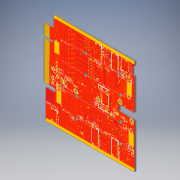
# Autodesk Inventor part: EPS_PCB
Saved by Autodesk Inventor 2018 (Build 220112000, 112)
## iProperties
Created: 2018-01-15
Part Number: EPS_PCB
Material: Epoxy Resin
Document SubType Name: Modeling
Designer: Bradley
Density: 1.14 g/cm^3
Appearance: Smooth - Medium Gray
Mass: 15.4834 g
Surface Area: 175.95 cm^2
Volume: 13.582 cm^3
Author: Bradley
Revision Number: 3.1
Autodesk Inventor part; units mm, degrees
ref_plane "YZ Plane" through (0, 0, 0) normal (1, 0, 0) x (0, 1, 0)
ref_plane "XZ Plane" through (0, 0, 0) normal (0, 1, 0) x (-1, 0, 0)
ref_plane "XY Plane" through (0, 0, 0) normal (0, 0, 1) x (1, 0, 0)
sketch "Sketch1" plane through (0, 0, 0) normal (0, 0, 1) x (1, 0, 0)
  line L0 (0, 36.15) -> (10, 36.15)
  line L1 (10, 36.15) -> (10, 47.9)
  line L2 (10, 47.9) -> (90.4, 47.9)
  line L3 (90.4, 47.9) -> (90.4, -47.9)
  line L4 (90.4, -47.9) -> (2, -47.9)
  line L5 (10, -15.15) -> (0, -15.15)
  line L6 (-5.5, 48) -> (90.5, 48) construction
  line L7 (90.5, 48) -> (90.5, -48) construction
  line L8 (90.5, -48) -> (-5.5, -48) construction
  line L9 (-5.5, -48) -> (-5.5, 48) construction
  line L10 (-5.4, 47.9) -> (-3.4, 47.9) construction
  line L11 (-3.4, 47.9) -> (-3.4, -47.9) construction
  line L12 (-3.4, -47.9) -> (-5.4, -47.9) construction
  line L13 (-5.4, -47.9) -> (-5.4, 47.9) construction
  line L14 (-3.4, 38.5) -> (7.85, 38.5) construction
  line L15 (7.85, 38.5) -> (7.85, -17.5) construction
  line L16 (7.85, -17.5) -> (-3.4, -17.5) construction
  line L17 (-3.4, -17.5) -> (-3.4, 38.5) construction
  line L18 (2, -47.9) -> (2, -18.65)
  line L19 (2, -18.65) -> (10, -18.65)
  arc A0 (10, -18.65) -> (10, -15.15) centre (10, -16.9) ccw
  line L20 (0, 24) -> (90.5, 24) construction
  circle A1 centre (-2.5, 47.1) radius 0.9 construction
  circle A2 centre (-0.7, 47.1) radius 0.9 construction
  circle A3 centre (1.1, 47.1) radius 0.9 construction
  circle A4 centre (2.9, 47.1) radius 0.9 construction
  circle A5 centre (4.7, 47.1) radius 0.9 construction
  circle A6 centre (6.5, 47.1) radius 0.9 construction
  circle A7 centre (8.3, 47.1) radius 0.9 construction
  circle A8 centre (-2.5, 45.3) radius 0.9 construction
  circle A9 centre (-0.7, 45.3) radius 0.9 construction
  circle A10 centre (1.1, 45.3) radius 0.9 construction
  circle A11 centre (2.9, 45.3) radius 0.9 construction
  circle A12 centre (4.7, 45.3) radius 0.9 construction
  circle A13 centre (6.5, 45.3) radius 0.9 construction
  circle A14 centre (8.3, 45.3) radius 0.9 construction
  circle A15 centre (-2.5, 43.5) radius 0.9 construction
  circle A16 centre (-0.7, 43.5) radius 0.9 construction
  circle A17 centre (1.1, 43.5) radius 0.9 construction
  circle A18 centre (2.9, 43.5) radius 0.9 construction
  circle A19 centre (4.7, 43.5) radius 0.9 construction
  circle A20 centre (6.5, 43.5) radius 0.9 construction
  circle A21 centre (8.3, 43.5) radius 0.9 construction
  circle A22 centre (-2.5, 41.7) radius 0.9 construction
  circle A23 centre (-0.7, 41.7) radius 0.9 construction
  circle A24 centre (1.1, 41.7) radius 0.9 construction
  circle A25 centre (2.9, 41.7) radius 0.9 construction
  circle A26 centre (4.7, 41.7) radius 0.9 construction
  circle A27 centre (6.5, 41.7) radius 0.9 construction
  circle A28 centre (8.3, 41.7) radius 0.9 construction
  circle A29 centre (-2.5, 39.9) radius 0.9 construction
  circle A30 centre (-0.7, 39.9) radius 0.9 construction
  circle A31 centre (1.1, 39.9) radius 0.9 construction
  circle A32 centre (2.9, 39.9) radius 0.9 construction
  circle A33 centre (4.7, 39.9) radius 0.9 construction
  circle A34 centre (6.5, 39.9) radius 0.9 construction
  circle A35 centre (8.3, 39.9) radius 0.9 construction
  line L21 (0, 36.15) -> (0, 24.95)
  line L22 (0, 24.95) -> (8.4, 24.95)
  arc A36 (8.4, 23.05) -> (8.4, 24.95) centre (8.4, 24) ccw
  line L23 (8.4, 23.05) -> (0, 23.05)
  line L24 (0, 23.05) -> (0, -15.15)
  point P0 (0, 0)
  point P1 (-5.5, 0)
  point P2 (90.4, 0)
  point P3 (90.5, 0)
  dimension "d0" = 51.3
  dimension "d1" = 95.8
  dimension "d3" = 10
  dimension "d20" = 96
  dimension "d21" = 96
  dimension "d22" = 0.1
  dimension "d23" = 0.1
  dimension "d24" = 2
  dimension "d25" = 0.1
  dimension "d28" = 11.25
  dimension "d29" = 56
  dimension "d31" = 9.5
  dimension "d32" = 30.5
  dimension "d34" = 3.5
  dimension "d35" = 12.15
  dimension "d36" = 39.15
  dimension "d37" = 14.5
  dimension "d38" = 1.15
  dimension "d39" = 1.8
  dimension "d42" = 1.8
  dimension "d45" = 1.8
  dimension "d48" = 2
  dimension "d49" = 3.4
  dimension "d50" = 1.9
  dimension "d51" = 8.4
  dimension "d52" = 24
  constraints: 50 end point, 37 centre point, 11 perpendicular, 7 parallel, 6 point on line, 6 tangent, 5 horizontal, 4 point on circle, 3 midpoint, 3 vertical, 2 collinear, 2 horizontal alignment, 68 other
  measures "d0" distance of L5.end L0.start
  measures "d1" distance of L2.end L3.end
  measures "d3" distance of L0.start L0.end
  measures "d20" distance of L6.start L6.end
  measures "d21" distance of L8.end L6.start
  measures "d22" distance between parallel lines of L2 L6
  measures "d23" distance between parallel lines of L7 L3
  measures "d24" distance between parallel lines of L13 L11
  measures "d25" distance between parallel lines of L13 L9
  measures "d28" distance of L15.end L16.end
  measures "d29" distance of L14.end L15.end
  measures "d31" distance between parallel lines of L14 L6
  measures "d32" distance between parallel lines of L8 L16
  measures "d34" distance between parallel lines of L5 L19
  measures "d35" distance between parallel lines of L20 L0
  measures "d36" distance between parallel lines of L5 L20
  measures "d37" distance between parallel lines of L20 L14
  measures "d38" distance between parallel lines of L19 L16
  measures "d39" diameter of A1
  measures "d42" distance of A1.centre A2.centre
  measures "d45" distance of A1.centre A8.centre
  measures "d48" distance between parallel lines of L18 L24
  measures "d49" distance between parallel lines of L24 L11
  measures "d50" distance between parallel lines of L23 L22
  measures "d51" distance of L21.end L22.end
  measures "d52" distance from line of point (0, 0) L20
extrude "Extrusion1" add sketch "Sketch1" along normal mid plane 1.6
chamfer "Chamfer1" distance 0.5 angle 45 4 edges at (0, 36.15, 0) (0, 24.95, 0) (0, 23.05, 0) (0, -15.15, 0)
fillet "Fillet1" radius 0.5 6 edges at (10, 36.15, 0) (10, 47.9, 0) (90.4, 47.9, 0) (90.4, -47.9, 0) (2, -47.9, 0) (2, -18.65, 0)
sketch "Sketch6" plane through (0, 0, 0.8) normal (0, 0, 1) x (1, 0, 0)
  arc A0 (2.5, -18.65) -> (2, -19.15) centre (2.5, -19.15) ccw projected
  line L0 (2, -19.15) -> (2, -47.4) projected
  arc A1 (2, -47.4) -> (2.5, -47.9) centre (2.5, -47.4) ccw projected
  line L1 (2.5, -47.9) -> (89.9, -47.9) projected
  arc A2 (89.9, -47.9) -> (90.4, -47.4) centre (89.9, -47.4) ccw projected
  line L2 (90.4, -47.4) -> (90.4, 47.4) projected
  arc A3 (90.4, 47.4) -> (89.9, 47.9) centre (89.9, 47.4) ccw projected
  line L3 (89.9, 47.9) -> (10.5, 47.9) projected
  arc A4 (10.5, 47.9) -> (10, 47.4) centre (10.5, 47.4) ccw projected
  line L4 (10, 47.4) -> (10, 36.65) projected
  arc A5 (9.5, 36.15) -> (10, 36.65) centre (9.5, 36.65) ccw projected
  line L5 (9.5, 36.15) -> (0.5, 36.15) projected
  line L6 (0, 35.65) -> (0.5, 36.15) projected
  line L7 (0, 35.65) -> (0, 25.45) projected
  line L8 (0.5, 24.95) -> (0, 25.45) projected
  line L9 (0.5, 24.95) -> (8.4, 24.95) projected
  arc A6 (8.4, 23.05) -> (8.4, 24.95) centre (8.4, 24) ccw projected
  line L10 (8.4, 23.05) -> (0.5, 23.05) projected
  line L11 (0, 22.55) -> (0.5, 23.05) projected
  line L12 (0, 22.55) -> (0, -14.65) projected
  line L13 (0.5, -15.15) -> (0, -14.65) projected
  line L14 (0.5, -15.15) -> (10, -15.15) projected
  arc A7 (10, -18.65) -> (10, -15.15) centre (10, -16.9) ccw projected
  line L15 (10, -18.65) -> (2.5, -18.65) projected
  line L16 (90.4, 47.4) -> (90.4, -47.4) projected
  arc A8 (89.4, 3) -> (90.4, 4) centre (89.4, 4) ccw
  line L17 (89.4, 3) -> (75.9, 3)
  arc A9 (75.9, 3) -> (74.9, 2) centre (75.9, 2) ccw
  line L18 (74.9, 2) -> (74.9, -2)
  arc A10 (74.9, -2) -> (75.9, -3) centre (75.9, -2) ccw
  line L19 (75.9, -3) -> (89.4, -3)
  arc A11 (90.4, -4) -> (89.4, -3) centre (89.4, -4) ccw
  arc A12 (90.4, 34) -> (89.4, 35) centre (89.4, 34) ccw
  arc A13 (88.4, 36) -> (89.4, 35) centre (89.4, 36) ccw
  line L20 (88.4, 36) -> (88.4, 42)
  arc A14 (89.4, 43) -> (88.4, 42) centre (89.4, 42) ccw
  arc A15 (89.4, 43) -> (90.4, 44) centre (89.4, 44) ccw
  point P0 (0, 0)
  point P1 (74.9, 0)
  dimension "d69" = 6
  dimension "d70" = 1
  dimension "d71" = 15.5
  dimension "d81" = 2
  dimension "d82" = 35
  dimension "d83" = 8
  constraints: 16 point on circle, 14 tangent, 8 centre point, 8 end point, 6 equal radius, 4 point on line, 2 perpendicular, 1 horizontal, 1 horizontal alignment, 1 midpoint, 1 vertical, 1 vertical alignment
  measures "d69" distance between parallel lines of L19 L17
  measures "d70" radius of A8
  measures "d71" distance between parallel lines of L2 L18
  measures "d81" distance between parallel lines of L16 L20
  measures "d82" vertical distance of point (0, 0) A12.end
  measures "d83" distance of A12.end A14.start
extrude "Extrusion5" cut sketch "Sketch6" against normal through all contours A11 L19 A10 L18 A9 L17 A8 L2 | A12 A13 L20 A14 A15 L2
sketch "Sketch14" plane through (0, 0, 0.8) normal (0, 0, 1) x (1, 0, 0)
  line L0 (0, 22.55) -> (0, -14.65) projected
  line L1 (90.4, 4) -> (90.4, 34) projected
  line L2 (0, 47.894) -> (90.4, 47.894) construction
  line L3 (90.4, 47.894) -> (90.4, -47.894) construction
  line L4 (90.4, -47.894) -> (0, -47.894) construction
  line L5 (0, -47.894) -> (0, 47.894) construction
  point P0 (0, 0)
  constraints: 1 collinear, 1 midpoint, 2 other
decal "Decal1"
sketch "Sketch15" plane through (0, 0, -0.8) normal (0, 0, -1) x (-1, 0, 0)
  line L0 (-90.4, 34) -> (-90.4, 4) projected
  line L1 (0, -14.65) -> (0, 22.55) projected
  line L2 (-90.4, 47.894) -> (0, 47.894) construction
  line L3 (0, 47.894) -> (0, -47.894) construction
  line L4 (0, -47.894) -> (-90.4, -47.894) construction
  line L5 (-90.4, -47.894) -> (-90.4, 47.894) construction
  point P0 (0, 0)
  constraints: 1 collinear, 1 midpoint, 2 other
decal "Decal2"
sketch "Sketch16" plane through (0, 0, 0.8) normal (0, 0, 1) x (1, 0, 0)
  point P0 (0, 0)
  point P1 (32.5, -11.5)
  point P2 (41.5, 30.5)
  point P3 (76, 30.5)
  point P4 (76, 11.5)
  point P5 (41.5, 11.5)
  point P6 (76, -11.5)
  point P7 (32.5, -30.5)
  point P8 (76, -30.5)
  constraints: 8 other
hole "Hole9" at (32.5, -11.5, 0.8) at (41.5, 30.5, 0.8) at (76, 30.5, 0.8) at (76, 11.5, 0.8) at (41.5, 11.5, 0.8) at (76, -11.5, 0.8) at (32.5, -30.5, 0.8) at (76, -30.5, 0.8) direction (0, 0, -1) diameter 3 end through all
sketch "Sketch17" plane through (0, 0, 0.8) normal (0, 0, 1) x (1, 0, 0)
  point P0 (0, 0)
  point P1 (75.9, 5.5)
  point P2 (54.3, -3.4)
  point P3 (87.4, -5.5)
  point P4 (31.9, -7.5)
  constraints: 4 other
hole "Hole10" at (75.9, 5.5, 0.8) at (54.3, -3.4, 0.8) at (87.4, -5.5, 0.8) at (31.9, -7.5, 0.8) direction (0, 0, -1) diameter 2.2 end through all
sketch "Sketch18" plane through (0, 0, 0.8) normal (0, 0, 1) x (1, 0, 0)
  point P0 (0, 0)
  point P1 (67.3, -9.5)
  point P2 (9.6, 0.7)
  point P3 (13.7, -4.1)
  point P4 (73.1, -5.9)
  constraints: 4 other
hole "Hole11" at (67.3, -9.5, 0.8) at (9.6, 0.7, 0.8) at (13.7, -4.1, 0.8) at (73.1, -5.9, 0.8) direction (0, 0, -1) diameter 1.5 end through all
sketch "Sketch19" plane through (0, 0, 0.8) normal (0, 0, 1) x (1, 0, 0)
  point P0 (0, 0)
  point P1 (57.46, 8)
  point P2 (62.54, 8)
  point P3 (62.54, -8)
  point P4 (57.46, -8)
  constraints: 4 other
hole "Hole12" at (57.46, 8, 0.8) at (62.54, 8, 0.8) at (62.54, -8, 0.8) at (57.46, -8, 0.8) direction (0, 0, -1) diameter 1.2 end through all
sketch "Sketch20" plane through (0, 0, 0.8) normal (0, 0, 1) x (1, 0, 0)
  point P0 (0, 0)
  point P1 (87.975, 4.15)
  point P2 (80.725, 4.15)
  point P3 (30.4, -3.2)
  constraints: 3 other
hole "Hole13" at (87.975, 4.15, 0.8) at (80.725, 4.15, 0.8) at (30.4, -3.2, 0.8) direction (0, 0, -1) diameter 0.7 end through all
sketch "Sketch21" plane through (0, 0, 0.8) normal (0, 0, 1) x (1, 0, 0)
  point P0 (0, 0)
  point P1 (74.769, 6.631)
  point P2 (74.3, 5.5)
  point P3 (74.769, 4.369)
  point P4 (75.9, 3.9)
  point P5 (77.031, 4.369)
  point P6 (89, -5.5)
  point P7 (88.531, -4.369)
  point P8 (86.269, -4.369)
  point P9 (30.769, -6.369)
  point P10 (30.3, -7.5)
  point P11 (30.769, -8.631)
  point P12 (31.9, -9.1)
  point P13 (33.031, -8.631)
  point P14 (88.531, -6.631)
  point P15 (55.9, -3.4)
  point P16 (55.431, -2.269)
  point P17 (54.3, -1.8)
  point P18 (53.169, -2.269)
  point P19 (52.7, -3.4)
  point P20 (87.4, -7.1)
  point P21 (54.3, -5)
  point P22 (55.431, -4.531)
  point P23 (33.5, -7.5)
  point P24 (33.031, -6.369)
  point P25 (31.9, -5.9)
  point P26 (87.4, -3.9)
  point P27 (77.5, 5.5)
  point P28 (77.031, 6.631)
  point P29 (75.9, 7.1)
  point P30 (86.269, -6.631)
  point P31 (85.8, -5.5)
  point P32 (53.169, -4.531)
  constraints: 32 other
hole "Hole14" at (74.769, 6.631, 0.8) at (74.3, 5.5, 0.8) at (74.769, 4.369, 0.8) at (75.9, 3.9, 0.8) at (77.031, 4.369, 0.8) at (89, -5.5, 0.8) at (88.531, -4.369, 0.8) at (86.269, -4.369, 0.8) at (30.769, -6.369, 0.8) at (30.3, -7.5, 0.8) at (30.769, -8.631, 0.8) at (31.9, -9.1, 0.8) at (33.031, -8.631, 0.8) at (88.531, -6.631, 0.8) at (55.9, -3.4, 0.8) at (55.431, -2.269, 0.8) at (54.3, -1.8, 0.8) at (53.169, -2.269, 0.8) at (52.7, -3.4, 0.8) at (87.4, -7.1, 0.8) at (54.3, -5, 0.8) at (55.431, -4.531, 0.8) at (33.5, -7.5, 0.8) at (33.031, -6.369, 0.8) at (31.9, -5.9, 0.8) at (87.4, -3.9, 0.8) at (77.5, 5.5, 0.8) at (77.031, 6.631, 0.8) at (75.9, 7.1, 0.8) at (86.269, -6.631, 0.8) at (85.8, -5.5, 0.8) at (53.169, -4.531, 0.8) direction (0, 0, -1) diameter 0.35 end through all
sketch "Sketch22" plane through (0, 0, 0.8) normal (0, 0, 1) x (1, 0, 0)
  point P0 (0, 0)
  point P1 (53.3, -21.6)
  point P2 (61.7, -27.3)
  point P3 (63.7, -24.1)
  point P4 (70.2, -35.2)
  point P5 (67.2, -35.2)
  point P6 (64.3, -35.2)
  point P7 (74.3, -34.5)
  point P8 (79.2, -31.9)
  point P9 (87.7, -11.7)
  point P10 (89.5, -7.5)
  point P11 (74.83, 21.6)
  point P12 (66.5, 32.5)
  point P13 (77, 26.5)
  point P14 (43.5, -36)
  point P15 (46.5, -36)
  point P16 (84, -31.5)
  point P17 (72.5, -26.5)
  point P18 (6, 13.5)
  point P19 (6, 12.5)
  point P20 (6, 11.5)
  point P21 (11.75, 44.15)
  point P22 (13.4, 40.05)
  point P23 (13.4, 35.95)
  point P24 (11.75, 31.7)
  point P25 (13.4, 11.35)
  point P26 (13.4, 7.25)
  point P27 (10.9, 2.25)
  point P28 (13.4, 15.35)
  point P29 (9.94, 19.885)
  point P30 (11.85, 26.56)
  point P31 (11.7, 29.55)
  point P32 (9.94, 21.51)
  point P33 (36.8, 43.65)
  point P34 (36.8, 6.85)
  point P35 (36.8, 15.25)
  point P36 (36.8, 19.15)
  point P37 (36.8, 23.25)
  point P38 (36.8, 27.35)
  point P39 (36.8, 31.45)
  point P40 (36.8, 35.55)
  point P41 (36.8, 39.65)
  point P42 (36.8, 10.95)
  point P43 (42.38, 43.68)
  point P44 (41.1, 38.3)
  point P45 (41.8, 35.5)
  point P46 (45.8, 43.7)
  point P47 (44.4, 41.1)
  point P48 (41.1, 41.1)
  point P49 (44.4, 38.3)
  point P50 (45.1, 35.5)
  point P51 (44.9, 26)
  point P52 (44.9, 23.2)
  point P53 (48.2, 26)
  point P54 (48.2, 23.2)
  point P55 (48.2, 20.4)
  point P56 (44.9, 20.4)
  point P57 (44.9, 17.6)
  point P58 (48.2, 17.6)
  point P59 (44.9, 14.8)
  point P60 (44.9, 12)
  point P61 (48.2, 12)
  point P62 (48.2, 14.8)
  point P63 (51.6, 42.7)
  point P64 (54.8, 22.2)
  point P65 (55.2, 25.6)
  point P66 (53.9, 30.9)
  point P67 (46.7, 35.5)
  point P68 (70, 43.8)
  point P69 (62.8, 43.8)
  point P70 (73.5, 33)
  point P71 (56.4, 43.8)
  point P72 (77.3, 43.8)
  point P73 (83.7, 43.8)
  point P74 (56.1, 33)
  point P75 (54.8, 15)
  point P76 (29.2, -11.9)
  point P77 (53, 0.9)
  point P78 (37.2, -16.9)
  point P79 (37.2, -17.6)
  point P80 (37.2, -18.3)
  point P81 (36.1, -9.8)
  point P82 (36.1, -10.6)
  point P83 (36.7, -4.5)
  point P84 (37.5, -4.5)
  point P85 (31.4, -2.5)
  point P86 (31.4, -3.9)
  point P87 (47.9, 1.5)
  point P88 (47.9, 2.2)
  point P89 (47.9, 0.8)
  point P90 (47.9, 0.1)
  point P91 (47.9, 2.9)
  point P92 (49.5, -7.2)
  point P93 (47.6, -9.1)
  point P94 (89.5, 7.1)
  point P95 (73.15, 1.2)
  point P96 (82.02, -6.1)
  point P97 (65.3, 9.1)
  point P98 (64.8, 13.6)
  point P99 (59.6, 12.4)
  point P100 (68.075, 9.1)
  point P101 (47.8, 7.6)
  point P102 (54.2, -42.5)
  point P103 (73.5, -40.5)
  point P104 (61.4, -42.7)
  point P105 (67.8, -42.7)
  point P106 (80.6, -42.6)
  point P107 (87.2, -42.3)
  point P108 (75.3, -38.1)
  point P109 (12.1, -41.3)
  point P110 (88.5, 9.7)
  point P111 (84.6, -3.9)
  point P112 (49.7, -18.8)
  point P113 (63.9, -16.1)
  point P114 (64.2, -18.8)
  point P115 (39, 6)
  point P116 (59.5, -8)
  point P117 (59, -3)
  point P118 (85, 39)
  point P119 (75.15, 23.135)
  point P120 (78.2, -34.2)
  point P121 (74.5, -33.75)
  point P122 (75.15, 22.375)
  point P123 (78.2, -35)
  point P124 (74.5, -35.25)
  point P125 (62.3, -1.2)
  point P126 (78.3, -20.9)
  point P127 (64.4, -11.5)
  point P128 (62.1, 42.2)
  point P129 (56.3, 40.5)
  point P130 (70.1, 42.2)
  point P131 (80.2, 39.6)
  point P132 (74.4, 42.5)
  point P133 (83, 39.6)
  point P134 (61.405, -44.41)
  point P135 (65.8, -35.2)
  point P136 (55, -44.1)
  point P137 (63, -35.2)
  point P138 (72.6, -43)
  point P139 (68.7, -35.2)
  point P140 (74.2, -43.1)
  point P141 (71.5, -35.2)
  point P142 (83.065, 30.67)
  point P143 (24.6, -40.3)
  point P144 (75.15, 23.895)
  point P145 (74.5, -32.2)
  point P146 (80.1, -33.1)
  point P147 (31.9, 20.8)
  point P148 (31.9, 24.9)
  point P149 (31.9, 29)
  point P150 (31.9, 33.1)
  point P151 (31.9, 37.2)
  point P152 (31.9, 41.3)
  point P153 (27.5, 43.095)
  point P154 (27.5, 39)
  point P155 (27.5, 34.9)
  point P156 (27.5, 30.8)
  point P157 (27.5, 26.7)
  point P158 (27.5, 22.6)
  point P159 (27.5, 18.5)
  point P160 (20.7, -14.4)
  point P161 (20.7, -11.3)
  point P162 (47.5, 37.6)
  point P163 (50.7, 17)
  point P164 (50.7, 9.8)
  point P165 (58.3, 33.7)
  point P166 (69.8, 38)
  point P167 (74.4, 25.6)
  point P168 (57.5, 26.7)
  point P169 (76.8, 34.7)
  point P170 (34.2, 2.5)
  point P171 (34.2, 1.9)
  point P172 (34.2, 1.2)
  point P173 (34.9, 1.2)
  point P174 (35.6, 1.2)
  point P175 (69.66, 22.7)
  point P176 (79, 21.6)
  point P177 (19.85, -5.4)
  point P178 (17.595, -8.33)
  point P179 (57.2, -20.8)
  point P180 (76.8, -15.1)
  point P181 (76, -37)
  point P182 (79.2, -36.1)
  point P183 (72.2, -36.5)
  point P184 (61.2, -38.2)
  point P185 (48.5, -28.5)
  point P186 (54.7, -25.3)
  point P187 (31.8, -43)
  point P188 (26.7, -41.5)
  point P189 (66.87, 37.495)
  point P190 (27.5, -35.6)
  point P191 (67.86, -22.24)
  point P192 (76.61, -22.88)
  point P193 (86.4, -26.1)
  point P194 (27.9, -13.1)
  point P195 (54.205, -20.385)
  point P196 (45.7, -14.3)
  point P197 (14.6, 1.8)
  point P198 (14.8, 2.8)
  point P199 (82.3, 20.5)
  constraints: 613 other
hole "Hole15" at (53.3, -21.6, 0.8) at (61.7, -27.3, 0.8) at (63.7, -24.1, 0.8) at (70.2, -35.2, 0.8) at (67.2, -35.2, 0.8) at (64.3, -35.2, 0.8) at (74.3, -34.5, 0.8) at (79.2, -31.9, 0.8) at (87.7, -11.7, 0.8) at (89.5, -7.5, 0.8) at (74.83, 21.6, 0.8) at (66.5, 32.5, 0.8) at (77, 26.5, 0.8) at (43.5, -36, 0.8) at (46.5, -36, 0.8) at (84, -31.5, 0.8) at (72.5, -26.5, 0.8) at (6, 13.5, 0.8) at (6, 12.5, 0.8) at (6, 11.5, 0.8) at (11.75, 44.15, 0.8) at (13.4, 40.05, 0.8) at (13.4, 35.95, 0.8) at (11.75, 31.7, 0.8) at (13.4, 11.35, 0.8) at (13.4, 7.25, 0.8) at (10.9, 2.25, 0.8) at (13.4, 15.35, 0.8) at (9.94, 19.885, 0.8) at (11.85, 26.56, 0.8) at (11.7, 29.55, 0.8) at (9.94, 21.51, 0.8) at (36.8, 43.65, 0.8) at (36.8, 6.85, 0.8) at (36.8, 15.25, 0.8) at (36.8, 19.15, 0.8) at (36.8, 23.25, 0.8) at (36.8, 27.35, 0.8) at (36.8, 31.45, 0.8) at (36.8, 35.55, 0.8) at (36.8, 39.65, 0.8) at (36.8, 10.95, 0.8) at (42.38, 43.68, 0.8) at (41.1, 38.3, 0.8) at (41.8, 35.5, 0.8) at (45.8, 43.7, 0.8) at (44.4, 41.1, 0.8) at (41.1, 41.1, 0.8) at (44.4, 38.3, 0.8) at (45.1, 35.5, 0.8) direction (0, 0, -1) diameter 0.3 end through all and at (44.9, 26, 0.8) (44.9, 23.2, 0.8) (48.2, 26, 0.8) (48.2, 23.2, 0.8) (48.2, 20.4, 0.8) (44.9, 20.4, 0.8) (44.9, 17.6, 0.8) (48.2, 17.6, 0.8) (44.9, 14.8, 0.8) (44.9, 12, 0.8) (48.2, 12, 0.8) (48.2, 14.8, 0.8) (51.6, 42.7, 0.8) (54.8, 22.2, 0.8) (55.2, 25.6, 0.8) (53.9, 30.9, 0.8) (46.7, 35.5, 0.8) (70, 43.8, 0.8) (62.8, 43.8, 0.8) (73.5, 33, 0.8) (56.4, 43.8, 0.8) (77.3, 43.8, 0.8) (83.7, 43.8, 0.8) (56.1, 33, 0.8) (54.8, 15, 0.8) (29.2, -11.9, 0.8) (53, 0.9, 0.8) (37.2, -16.9, 0.8) (37.2, -17.6, 0.8) (37.2, -18.3, 0.8) (36.1, -9.8, 0.8) (36.1, -10.6, 0.8) (36.7, -4.5, 0.8) (37.5, -4.5, 0.8) (31.4, -2.5, 0.8) (31.4, -3.9, 0.8) (47.9, 1.5, 0.8) (47.9, 2.2, 0.8) (47.9, 0.8, 0.8) (47.9, 0.1, 0.8) (47.9, 2.9, 0.8) (49.5, -7.2, 0.8) (47.6, -9.1, 0.8) (89.5, 7.1, 0.8) (73.15, 1.2, 0.8) (82.02, -6.1, 0.8) (65.3, 9.1, 0.8) (64.8, 13.6, 0.8) (59.6, 12.4, 0.8) (68.075, 9.1, 0.8) (47.8, 7.6, 0.8) (54.2, -42.5, 0.8) (73.5, -40.5, 0.8) (61.4, -42.7, 0.8) (67.8, -42.7, 0.8) (80.6, -42.6, 0.8) (87.2, -42.3, 0.8) (75.3, -38.1, 0.8) (12.1, -41.3, 0.8) (88.5, 9.7, 0.8) (84.6, -3.9, 0.8) (49.7, -18.8, 0.8) (63.9, -16.1, 0.8) (64.2, -18.8, 0.8) (39, 6, 0.8) (59.5, -8, 0.8) (59, -3, 0.8) (85, 39, 0.8) (75.15, 23.135, 0.8) (78.2, -34.2, 0.8) (74.5, -33.75, 0.8) (75.15, 22.375, 0.8) (78.2, -35, 0.8) (74.5, -35.25, 0.8) (62.3, -1.2, 0.8) (78.3, -20.9, 0.8) (64.4, -11.5, 0.8) (62.1, 42.2, 0.8) (56.3, 40.5, 0.8) (70.1, 42.2, 0.8) (80.2, 39.6, 0.8) (74.4, 42.5, 0.8) (83, 39.6, 0.8) (61.405, -44.41, 0.8) (65.8, -35.2, 0.8) (55, -44.1, 0.8) (63, -35.2, 0.8) (72.6, -43, 0.8) (68.7, -35.2, 0.8) (74.2, -43.1, 0.8) (71.5, -35.2, 0.8) (83.065, 30.67, 0.8) (24.6, -40.3, 0.8) (75.15, 23.895, 0.8) (74.5, -32.2, 0.8) (80.1, -33.1, 0.8) (31.9, 20.8, 0.8) (31.9, 24.9, 0.8) (31.9, 29, 0.8) (31.9, 33.1, 0.8) (31.9, 37.2, 0.8) (31.9, 41.3, 0.8) (27.5, 43.095, 0.8) (27.5, 39, 0.8) (27.5, 34.9, 0.8) (27.5, 30.8, 0.8) (27.5, 26.7, 0.8) (27.5, 22.6, 0.8) (27.5, 18.5, 0.8) (20.7, -14.4, 0.8) (20.7, -11.3, 0.8) (47.5, 37.6, 0.8) (50.7, 17, 0.8) (50.7, 9.8, 0.8) (58.3, 33.7, 0.8) (69.8, 38, 0.8) (74.4, 25.6, 0.8) (57.5, 26.7, 0.8) (76.8, 34.7, 0.8) (34.2, 2.5, 0.8) (34.2, 1.9, 0.8) (34.2, 1.2, 0.8) (34.9, 1.2, 0.8) (35.6, 1.2, 0.8) (69.66, 22.7, 0.8) (79, 21.6, 0.8) (19.85, -5.4, 0.8) (17.595, -8.33, 0.8) (57.2, -20.8, 0.8) (76.8, -15.1, 0.8) (76, -37, 0.8) (79.2, -36.1, 0.8) (72.2, -36.5, 0.8) (61.2, -38.2, 0.8) (48.5, -28.5, 0.8) (54.7, -25.3, 0.8) (31.8, -43, 0.8) (26.7, -41.5, 0.8) (66.87, 37.495, 0.8) (27.5, -35.6, 0.8) (67.86, -22.24, 0.8) (76.61, -22.88, 0.8) (86.4, -26.1, 0.8) (27.9, -13.1, 0.8) (54.205, -20.385, 0.8) (45.7, -14.3, 0.8) (14.6, 1.8, 0.8) (14.8, 2.8, 0.8) (82.3, 20.5, 0.8) (77.56, 23.685, 0.8) (27.5, -0.5, 0.8) (57.5, 3.4, 0.8) (11.9, 2.8, 0.8) (30.1, -35.6, 0.8) (42.4, 42.6, 0.8) (42.4, 39.8, 0.8) (42.4, 37, 0.8) (43.1, 34.2, 0.8) (45.7, 36.9, 0.8) (45.7, 39.7, 0.8) (45.7, 42.5, 0.8) (46.2, 24.7, 0.8) (46.2, 21.9, 0.8) (46.2, 19.1, 0.8) (46.2, 16.3, 0.8) (49.5, 24.7, 0.8) (49.5, 21.9, 0.8) (49.5, 19.1, 0.8) (49.5, 16.3, 0.8) (46.14, 13.46, 0.8) (46.2, 10.7, 0.8) (49.5, 10.7, 0.8) (49.46, 13.85, 0.8) (57.2, 19.3, 0.8) (54, 39.9, 0.8) (84, 35.6, 0.8) (57.2, 12.1, 0.8) (87.7, 31.1, 0.8) (87.96, 22.3, 0.8) (63.58, 22.785, 0.8) (50.6, 7.6, 0.8) (82.04, 16.04, 0.8) (81.245, 16.835, 0.8) (51.775, 6.2, 0.8) (84, -16.3, 0.8) (75.63, -5.375, 0.8) (79.1, -5.5, 0.8) (60.5, -26.1, 0.8) (66.7, -26.4, 0.8) (57.9, -19.175, 0.8) (75.5, -15.075, 0.8) (47.5, -25.3, 0.8) (37.2, -20.6, 0.8) (38.3, -22.3, 0.8) (35.4, -30.2, 0.8) (23.8, -42.9, 0.8) (35.6, -42.1, 0.8) (35.3, -36, 0.8) (88.5, 44.4, 0.8) (89.8, -44.4, 0.8) (87.96, 18.09, 0.8) (87.96, 18.855, 0.8) (85.53, 26.705, 0.8) (85.635, 28.785, 0.8) (84.335, 29.855, 0.8) (85.095, 29.82, 0.8) (87.2, -28.2, 0.8) (86.4, -28.2, 0.8) (89.4, -29.1, 0.8) (87.2, -13, 0.8) (86.4, -13, 0.8) (15.5, -9.6, 0.8) (17.6, -11.9, 0.8) (28.1, -34.4, 0.8) (89.4, -31.2, 0.8) (85.7, 40.6, 0.8) (86.4, 40.6, 0.8) (82.4, 15.1, 0.8) (81.8, 14.8, 0.8) (82.4, 14.5, 0.8) (84.4, -15.1, 0.8) (84.4, -14.5, 0.8) (83.8, -14.8, 0.8) (67.12, -1.5, 0.8) (59.3, -43.8, 0.8) (65.7, -43.8, 0.8) (72.1, -43.8, 0.8) (78.5, -43.8, 0.8) (38, 0.8, 0.8) (27.6, -3, 0.8) (49.5, -20.9, 0.8) (6, 35.5, 0.8) (10.6, 42.65, 0.8) (20.86, -2.76, 0.8) (6, 34.5, 0.8) (11.36, 41.855, 0.8) (6, 33.5, 0.8) (12.12, 37.705, 0.8) (6, 32.5, 0.8) (6, 31.5, 0.8) (6, 30.5, 0.8) (6, 29.5, 0.8) (6, 28.5, 0.8) (6, 27.5, 0.8) (6, 26.5, 0.8) (6, 25.55, 0.8) (6, 22.45, 0.8) (6, 21.5, 0.8) (54.2, -17.31, 0.8) (68.5, -16.3, 0.8) (29.5, 33.4, 0.8) (21.3, -10.6, 0.8) (37.7, -35.4, 0.8) (33.6, -38.5, 0.8) (6, 20.5, 0.8) (6, 19.5, 0.8) (6, 18.5, 0.8) (6, 17.5, 0.8) (6, 16.5, 0.8) (6, 15.5, 0.8) (6, 14.5, 0.8) (7.71, 11.44, 0.8) (50.1, 12.5, 0.8) (48.6, 6.9, 0.8) (27.7, 44.3, 0.8) (31.48, -33.28, 0.8) (69.8, 33, 0.8) (43.38, -23.27, 0.8) (68.59, 36.29, 0.8) (42.195, -24.23, 0.8) (43.485, -25.06, 0.8) (9.3, -14.1, 0.8) (18.9, -11.6, 0.8) (18.65, -17.1, 0.8) (18.9, -14.3, 0.8) (6, -9.5, 0.8) (16.7, -6.52, 0.8) (6, -8.5, 0.8) (16.7, -4.385, 0.8) (6, -10.5, 0.8) (16.7, -7.28, 0.8) (70.59, 32.645, 0.8) (43.81, -24.37, 0.8) (70.6, 31, 0.8) (42.945, -24.37, 0.8) (6, -7.5, 0.8) (16.7, -3.62, 0.8) (51.6, 18, 0.8) (48.4, 38.6, 0.8) (51.6, 10.8, 0.8) (64.01, 30.295, 0.8) (50.66, 6.165, 0.8) (54.88, -20.8, 0.8) (56, -20.8, 0.8) (80.7, -36.64, 0.8) (29.655, -42.765, 0.8) (52.335, 17.8, 0.8) (49.135, 38.4, 0.8) (52.335, 10.6, 0.8) (64.01, 29.535, 0.8) (51.235, 5.665, 0.8) (55.5, -21.4, 0.8) (80.7, -32.56, 0.8) (30.41, -43.14, 0.8) (72.71, 30.325, 0.8) (72.7, 36, 0.8) (73.6, 19.995, 0.8) (42.7, -30, 0.8) (23.095, -4.08, 0.8) (57.82, 27.67, 0.8) (61.75, 27.75, 0.8) (76.725, -18.57, 0.8) (64.44, -6.33, 0.8) (73.685, -18.69, 0.8) (72.8, -19.505, 0.8) (62.29, 28.29, 0.8) (77.365, -18.16, 0.8) (64.76, -7.02, 0.8) (73.01, -18.335, 0.8) (73.34, -20.045, 0.8) (61.21, 28.79, 0.8) (61.21, 27.21, 0.8) (76.725, -19.33, 0.8) (64.12, -5.64, 0.8) (74.005, -19.38, 0.8) (61.97, 30.87, 0.8) (23.48, -5.945, 0.8) (61.98, 31.63, 0.8) (23.1, -4.84, 0.8) (61.21, 30.87, 0.8) (23.09, -6.6, 0.8) (74.93, -20.955, 0.8) (71.94, -20.965, 0.8) (45.63, -25.255, 0.8) (85.27, 35.61, 0.8) (84.015, -17.1, 0.8) (77.365, -19.74, 0.8) (75.645, -20.695, 0.8) (55.7, 44.4, 0.8) (57.2, 22.9, 0.8) (57.5, 14, 0.8) (63, -26.95, 0.8) (36.25, -39.59, 0.8) (68.3, -24.4, 0.8) (28.6, -32.1, 0.8) (75.385, -13.995, 0.8) (67.7, -18.8, 0.8) (86.58, 43.095, 0.8) (84.12, 11.84, 0.8) (76.26, -14.535, 0.8) (70.5, -17.5, 0.8) (68.54, -21.56, 0.8) (77.8, -21.9, 0.8) (82.9, 26.5, 0.8) (81.82, 26.265, 0.8) (82.9, 27.1, 0.8) (82.9, 27.7, 0.8) (83.5, 26.5, 0.8) (84.3, -27.7, 0.8) (84.3, -27.1, 0.8) (84.3, -26.5, 0.8) (83.7, -26.8, 0.8) (83.7, -27.4, 0.8) (72.4, -0.2, 0.8) (67.4, -0.2, 0.8) (67.4, -2.8, 0.8) (72.4, -2.8, 0.8) (72.15, 0.39, 0.8) (72.4, -3.5, 0.8) (67.4, 0.5, 0.8) (67.4, -3.5, 0.8) (11.9, 1.3, 0.8) (13.3, -8.7, 0.8) (62.3, 0.4, 0.8) (26.8, -2.4, 0.8) (31.9, 12.6, 0.8) (31.9, 8.5, 0.8) (31.9, 4.4, 0.8) (31.9, 16.7, 0.8) (27.5, 14.4, 0.8) (27.5, 10.3, 0.8) (27.5, 6.2, 0.8) (18.7, -26.9, 0.8) (42.5, -15.6, 0.8) (43.2, -15.6, 0.8) (43.9, -15.6, 0.8) (44.6, -15.6, 0.8) (44.6, -14.9, 0.8) (44.6, -14.2, 0.8) (78.9, 22.7, 0.8) (64.2, -12.7, 0.8) (63.5, -13.4, 0.8) (63.5, -14.1, 0.8) (63.5, -14.8, 0.8) (64.2, -14.8, 0.8) (64.2, -14.1, 0.8) (80.5, 31, 0.8) (63.5, -12.7, 0.8) (52.5, -9.2, 0.8) (60.7, -2.2, 0.8) (65.52, 7, 0.8) (74.265, -12.875, 0.8) (65.325, -10.88, 0.8) (74.005, -12.16, 0.8) (66.2, -14.8, 0.8) (66.9, -14.8, 0.8) (67.6, -14.8, 0.8) (68.3, -14.8, 0.8) (52.2, -5.3, 0.8) (50.2, -20.6, 0.8) (54.045, -18.055, 0.8) (65.1, -17.9, 0.8) (24.4, 42.2, 0.8) (40.6, 43.3, 0.8) (25.2, 42.2, 0.8) (40.6, 42.5, 0.8) (29.1, 40.4, 0.8) (43.9, 43.3, 0.8) (29.9, 40.4, 0.8) (43.9, 42.5, 0.8) (24.4, 38.1, 0.8) (40.6, 40.5, 0.8) (25.2, 38.1, 0.8) (40.6, 39.7, 0.8) (29.1, 36.3, 0.8) (43.9, 40.5, 0.8) (29.9, 36.3, 0.8) (43.9, 39.7, 0.8) (24.4, 34, 0.8) (40.6, 37.7, 0.8) (25.2, 34, 0.8) (40.6, 36.9, 0.8) (29.1, 32.2, 0.8) (43.9, 37.7, 0.8) (29.9, 32.2, 0.8) (43.9, 36.9, 0.8) (24.4, 29.9, 0.8) (41.3, 34.9, 0.8) (25.2, 29.9, 0.8) (41.6, 34.2, 0.8) (29.1, 28.1, 0.8) (44.6, 34.9, 0.8) (29.9, 28.1, 0.8) (44.6, 34.1, 0.8) (24.4, 25.8, 0.8) (44.4, 25.4, 0.8) (25.2, 25.8, 0.8) (44.4, 24.6, 0.8) (29.1, 24, 0.8) (47.7, 25.4, 0.8) (29.9, 24, 0.8) (47.7, 24.6, 0.8) (24.4, 21.7, 0.8) (44.4, 22.6, 0.8) (25.2, 21.7, 0.8) (44.4, 21.8, 0.8) (29.1, 19.9, 0.8) (47.7, 22.6, 0.8) (29.9, 19.9, 0.8) (47.7, 21.8, 0.8) (24.4, 17.6, 0.8) (44.4, 19.8, 0.8) (25.2, 17.6, 0.8) (44.4, 19, 0.8) (39.085, 32.235, 0.8) (46.7, 31.7, 0.8) (39.42, 30.81, 0.8) (45.2, 31.38, 0.8) (39.05, 31.475, 0.8) (45.965, 31.38, 0.8) (29.1, 15.8, 0.8) (47.7, 19.8, 0.8) (29.9, 15.8, 0.8) (47.7, 19, 0.8) (24.4, 13.5, 0.8) (44.4, 17, 0.8) (25.2, 13.5, 0.8) (44.4, 16.2, 0.8) (29.1, 11.7, 0.8) (64.2, -13.4, 0.8) (29.9, 11.7, 0.8) (47.7, 16.2, 0.8) (24.4, 9.4, 0.8) (44.4, 14.22, 0.8) (25.2, 9.4, 0.8) (44.425, 13.46, 0.8) (29.1, 7.6, 0.8) (47.7, 14.2, 0.8) (29.9, 7.6, 0.8) (47.7, 13.4, 0.8) (24.4, 5.3, 0.8) (44.4, 11.4, 0.8) (25.2, 5.3, 0.8) (44.4, 10.6, 0.8) (29.1, 3.5, 0.8) (47.7, 11.4, 0.8) (29.9, 3.5, 0.8) (47.7, 10.6, 0.8) (56.4, -9.2, 0.8) (14.3, -38.2, 0.8) (76.44, 25.045, 0.8) (74.275, 24.55, 0.8) (78.8, 31.2, 0.8) (79.5, 31.2, 0.8) (76.28, -16.825, 0.8) (70.57, -19.53, 0.8) (13, -37.5, 0.8) (17.1, -12.9, 0.8) (83.8, 32.2, 0.8) (30.7, 44.3, 0.8) (85.82, 43.095, 0.8) (83.1, 12.4, 0.8) (66.61, 38.21, 0.8) (82.9, -21, 0.8) (78.9, -21.4, 0.8) (80.44, -21.605, 0.8) (80.3, -24.4, 0.8) (74.87, -5.385, 0.8) (79.1, -6.3, 0.8) (64.3, -24.7, 0.8) (54.56, -18.615, 0.8) (58.4, -18.6, 0.8) (75.715, -15.805, 0.8) (68.62, -22.32, 0.8) (77.2, -22.4, 0.8) (48.2, -26.195, 0.8) (46.1, -22.3, 0.8) (51.9, -21.3, 0.8) (36.9, -22.1, 0.8) (33.41, -32.915, 0.8) (22.4, -16.6, 0.8) (22.4, -13.7, 0.8) (18.2, -11.3, 0.8) (50.5, 37.6, 0.8) (53.7, 17, 0.8) (58.3, 32.2, 0.8) (69, 38, 0.8) (74.4, 26.4, 0.8) (57.5, 25.9, 0.8) (65.7, 16.3, 0.8) (71, 16.8, 0.8) (53.7, 9.8, 0.8) (76.7, 35.5, 0.8) (64.11, 24.69, 0.8) (73.7, 21.6, 0.8) (16.59, -5.445, 0.8) (16.7, -2.8, 0.8) (55.1, 6.2, 0.8) (55.1, 5.6, 0.8) (79.7, -14.2, 0.8) (77.8, -10.4, 0.8) (58.4, -22.8, 0.8) (79.2, -33.1, 0.8) (54.7, -26.2, 0.8) (45.3, -31, 0.8) (26.7, -43.1, 0.8) (39.3, -27.6, 0.8) (33.1, -27.3, 0.8) (74.9, -23.5, 0.8) (70.9, -20.4, 0.8) (64.4, 33.1, 0.8) (52.6, 36.6, 0.8) (47.7, 17, 0.8)
equation "\"d23\" = d22"
equation "\"d25\" = d22"
equation "\"d42\" = d39"
equation "\"d45\" = d39"
body "Solid1"
